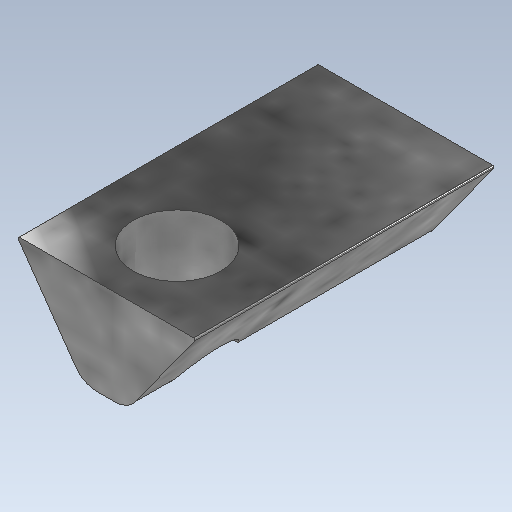
# Autodesk Inventor part: Tuerca
Saved by Autodesk Inventor 2021 (Build 250183000, 183)
## iProperties
Created: 2020-10-30
Part Number: Tuerca
Material: Acero, galvanizado
Document SubType Name: Modeling
Designer: juanm
Density: 7.85 g/cm^3
Appearance: Acero galvanizado
Author: juanm
Autodesk Inventor part; units mm, degrees
ref_plane "YZ Plane" through (0, 0, 0) normal (1, 0, 0) x (0, 1, 0)
ref_plane "XZ Plane" through (0, 0, 0) normal (0, 1, 0) x (-1, 0, 0)
ref_plane "XY Plane" through (0, 0, 0) normal (0, 0, 1) x (1, 0, 0)
sketch "Boceto1" plane through (0, 0, 0) normal (0, 0, 1) x (1, 0, 0)
  line L0 (0.1921, 0) -> (13.6079, 0)
  line L1 (0.1102, -0.1574) -> (4.514, -6.4466)
  line L2 (0, 0) -> (7.6778, 0) construction
  line L3 (6.1507, -7.2995) -> (6.8282, -7.3)
  arc A0 (0.1921, 0) -> (0.1102, -0.1574) centre (0.1921, -0.1) ccw
  arc A1 (13.6898, -0.1574) -> (13.6079, 0) centre (13.6079, -0.1) ccw
  line L4 (6.8282, 0) -> (6.8282, -7.3)
  line L5 (13.6898, -0.1574) -> (9.144, -6.4684)
  line L6 (7.5227, -7.2995) -> (6.8282, -7.3)
  arc A2 (7.5227, -7.2995) -> (9.144, -6.4684) centre (7.5211, -5.2995) ccw
  arc A3 (4.514, -6.4466) -> (6.1507, -7.2995) centre (6.1523, -5.2995) ccw
  point P0 (13.8, 0)
  point P1 (5.1106, -7.2986)
  point P2 (8.5459, -7.2986)
  dimension "d7" = 13.8
  dimension "d9" = 8.91
  dimension "d10" = 55
  dimension "d11" = 0.1
  dimension "d14" = 2
  dimension "d15" = 7.3
  constraints: 14 end point, 8 point on circle, 8 point on line, 7 tangent, 4 centre point, 2 equal radius, 2 horizontal, 1 equal length, 1 perpendicular, 1 symmetric about line
  measures "d7" distance of L2.start point (13.8, 0)
  measures "d9" distance of L2.start point (5.111, -7.299)
  measures "d10" angle of L1 L2
  measures "d11" radius of A0
  measures "d14" radius of A2
  measures "d15" distance of L4.start L3.end
extrude "Extrusión1" add sketch "Boceto1" along normal blind 23
sketch "Boceto2" plane through (0.1921, 0, 0) normal (0, 1, 0) x (1, 0, 0)
  circle A0 centre (6.6362, -17.5) radius 3.375
  point P0 (-0.1921, 0)
  point P1 (6.6362, -23)
  dimension "d17" = 6.75
  constraints: 1 centre point
  measures "d17" diameter of A0
extrude "Extrusión2" cut sketch "Boceto2" against normal blind 7.3
